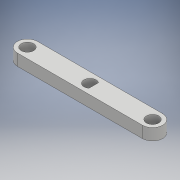
# Autodesk Inventor part: spinner
Saved by Autodesk Inventor 2018 (Build 220112000, 112)
## iProperties
Created: 2018-03-21
Part Number: spinner
Material: Generic
Document SubType Name: Modeling
Designer: Matt
Density: 1 g/cm^3
Appearance: Default
Author: Matt
Autodesk Inventor part; units mm, degrees
ref_plane "YZ Plane" through (0, 0, 0) normal (1, 0, 0) x (0, 1, 0)
ref_plane "XZ Plane" through (0, 0, 0) normal (0, 1, 0) x (-1, 0, 0)
ref_plane "XY Plane" through (0, 0, 0) normal (0, 0, 1) x (1, 0, 0)
sketch "Sketch1" plane through (0, 0, 0) normal (0, 0, 1) x (1, 0, 0)
  arc A0 (0.975, 1.2369) -> (0.975, -1.2369) centre (0, 0) ccw
  circle A1 centre (-16.2, 0) radius 1.6
  circle A2 centre (16.2, 0) radius 1.6
  arc A3 (-16.2, 2.6) -> (-16.2, -2.6) centre (-16.2, 0) ccw
  arc A4 (16.2, -2.6) -> (16.2, 2.6) centre (16.2, 0) ccw
  line L0 (16.2, 2.6) -> (-16.2, 2.6)
  line L1 (-16.2, -2.6) -> (16.2, -2.6)
  line L2 (0.975, 1.2369) -> (0.975, -1.2369)
  point P0 (-1.575, 0)
  dimension "d0" = 3.15
  dimension "d1" = 3.2
  dimension "d2" = 3.2
  dimension "d3" = 16.2
  dimension "d4" = 16.2
  dimension "d5" = 5.2
  dimension "d6" = 5.2
  dimension "d9" = 2.55
  constraints: 7 point on circle, 6 end point, 5 centre point, 3 coincident, 1 horizontal, 1 parallel, 1 tangent, 1 vertical
  measures "d0" diameter of A0
  measures "d1" diameter of A1
  measures "d2" diameter of A2
  measures "d3" distance of point (0, 0) A1.centre
  measures "d4" distance of A2.centre point (0, 0)
  measures "d5" diameter of A3
  measures "d6" diameter of A4
  measures "d9" distance from line of L2 point (-1.575, 0)
extrude "Extrusion1" add sketch "Sketch1" along normal blind 3
body "Solid1"
